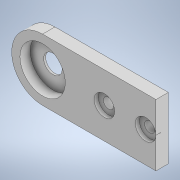
# Autodesk Inventor part: bearing_mount
Saved by Autodesk Inventor 2022.3 (Build 263350000, 350)
## iProperties
Created: 2022-01-28
Part Number: bearing_mount
Material: Generic
Document SubType Name: Modeling
Designer: Martijn
Density: 1 g/cm^3
Appearance: Default
Author: Martijn
Autodesk Inventor part; units mm, degrees
ref_plane "YZ Plane" through (0, 0, 0) normal (1, 0, 0) x (0, 1, 0)
ref_plane "XZ Plane" through (0, 0, 0) normal (0, 1, 0) x (-1, 0, 0)
ref_plane "XY Plane" through (0, 0, 0) normal (0, 0, 1) x (1, 0, 0)
sketch "Sketch1" plane through (0, 0, 0) normal (0, 0, 1) x (1, 0, 0)
  line L0 (15, 15) -> (70, 15)
  line L1 (70, 15) -> (70, -15)
  line L2 (70, -15) -> (15, -15)
  line L3 (-14, 0) -> (84, 0) projected
  arc A0 (15, 15) -> (15, -15) centre (15, 0) ccw
  line L4 (0, -21) -> (0, 21) projected
  line L5 (15, 0) -> (70, 0)
  point P0 (0, 0)
  dimension "d4" = 30
  dimension "d15" = 15
  dimension "d16" = 55
  constraints: 8 end point, 2 parallel, 2 point on circle, 1 centre point, 1 midpoint, 1 perpendicular, 1 point on line, 1 tangent, 1 vertical
  measures "d4" distance between parallel lines of L2 L0
  measures "d15" radius of A0
  measures "d16" distance from line of L1 L5.start
extrude "Extrusion1" add sketch "Sketch1" along normal blind 6
sketch "Sketch2" plane through (0, 0, 6) normal (0, 0, 1) x (1, 0, 0)
  circle A0 centre (15, 0) radius 11
  arc A1 (15, 15) -> (15, -15) centre (15, 0) ccw projected
  point P0 (0, 0)
  dimension "d7" = 22
  constraints: 1 centre point, 1 concentric
  measures "d7" diameter of A0
extrude "Extrusion2" cut sketch "Sketch2" against normal blind 10
sketch "Sketch3" plane through (0, 0, 6) normal (0, 0, 1) x (1, 0, 0)
  circle A0 centre (65, 0) radius 2.5
  line L0 (70, -15) -> (70, 15) projected
  circle A1 centre (45, 0) radius 2.5
  point P0 (0, 0)
  dimension "d10" = 5
  dimension "d12" = 5
  dimension "d26" = 5
  dimension "d27" = 20
  constraints: 2 centre point
  measures "d10" diameter of A0
  measures "d12" distance from line of L0 A0.centre
  measures "d26" diameter of A1
  measures "d27" distance of A0.centre A1.centre
extrude "Extrusion3" cut sketch "Sketch3" against normal blind 10
sketch "Sketch4" plane through (0, 0, 0) normal (0, 0, -1) x (-1, 0, 0)
  circle A0 centre (-15, 0) radius 15
  arc A1 (-15, -15) -> (-15, 15) centre (-15, 0) ccw projected
  circle A2 centre (-15, 0) radius 11 projected
  point P0 (0, 0)
  constraints: 2 concentric, 1 centre point
extrude "Extrusion4" add sketch "Sketch4" against normal blind 1 contours A0 | A2
sketch "Sketch6" plane through (0, 0, 6) normal (0, 0, 1) x (1, 0, 0)
  circle A0 centre (65, 0) radius 2.5 projected
  circle A1 centre (65, 0) radius 5
  circle A2 centre (45, 0) radius 5
  circle A3 centre (45, 0) radius 2.5 projected
  point P0 (0, 0)
  dimension "d22" = 10
  dimension "d28" = 10
  constraints: 2 centre point, 1 coincident, 1 concentric
  measures "d22" diameter of A1
  measures "d28" diameter of A2
extrude "Extrusion6" cut sketch "Sketch6" against normal blind 2
sketch "Sketch7" plane through (0, 0, 0) normal (0, 0, -1) x (-1, 0, 0)
  arc A0 (-15, -15) -> (-15, 15) centre (-15, 0) ccw projected
  circle A1 centre (-15, 0) radius 4.5
  point P0 (0, 0)
  dimension "d29" = 9
  constraints: 1 centre point, 1 coincident
  measures "d29" diameter of A1
extrude "Extrusion7" cut sketch "Sketch7" against normal blind 2
body "Solid1"
